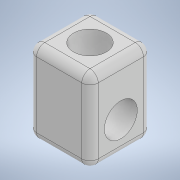
# Autodesk Inventor part: cantoneira
Saved by Autodesk Inventor 2022 (Build 260153000, 153)
## iProperties
Created: 2022-02-16
Part Number: cantoneira
Material: Genérico
Document SubType Name: Modeling
Designer: mathe
Density: 1 g/cm^3
Appearance: Padrão
Author: mathe
Autodesk Inventor part; units mm, degrees
ref_plane "YZ Plane" through (0, 0, 0) normal (1, 0, 0) x (0, 1, 0)
ref_plane "XZ Plane" through (0, 0, 0) normal (0, 1, 0) x (-1, 0, 0)
ref_plane "XY Plane" through (0, 0, 0) normal (0, 0, 1) x (1, 0, 0)
sketch "Esboço1" plane through (0, 0, 0) normal (0, 1, 0) x (-1, 0, 0)
  line L0 (0, 0) -> (15, 0)
  line L1 (15, 0) -> (15, -15)
  line L2 (15, -15) -> (0, -15)
  line L3 (0, -15) -> (0, 0)
  dimension "d0" = 15
  dimension "d1" = 15
  constraints: 8 end point, 2 parallel, 1 horizontal, 1 perpendicular
  measures "d0" distance of L1.end L2.end
  measures "d1" distance of L0.end L1.end
extrude "Extrusão1" add sketch "Esboço1" along normal blind 20
sketch "Esboço2" plane through (0, 0, 0) normal (1, 0, 0) x (0, 0, -1)
  point P0 (0, 0)
  point P1 (7.5, 7.5)
hole "Furo1" at (0, 7.5, -7.5) direction (-1, 0, 0) diameter 8 depth 12
sketch "Esboço4" plane through (0, 20, 0) normal (0, 1, 0) x (1, 0, 0)
  point P0 (0, 0)
  point P1 (-7.5, 7.5)
hole "Furo2" at (-7.5, 20, -7.5) direction (0, -1, 0) diameter 8 depth 7.5
fillet "Arredondamento1" radius 2 12 edges at (-7.5, 20, 0) (-15, 10, 0) (-15, 20, -7.5) (-7.5, 0, 0) (-15, 0, -7.5) (-15, 10, -15) (-7.5, 0, -15) (-7.5, 20, -15) (0, 10, -15) (0, 0, -7.5) (0, 10, 0) (0, 20, -7.5)
